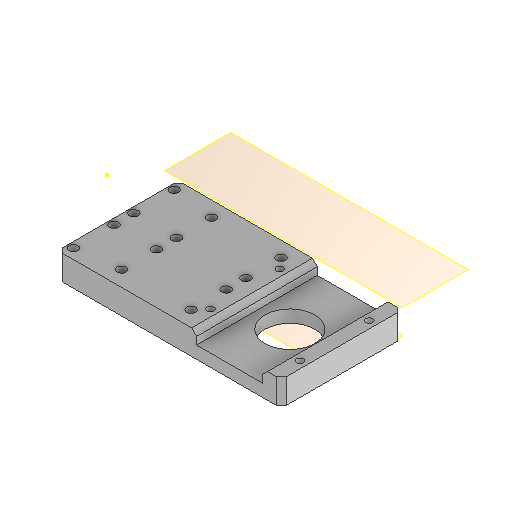
# Autodesk Inventor part: 60_Planktoscope_Sampleholder
Saved by Autodesk Inventor 2024.1 (Build 281209000, 209)
## iProperties
Created: 2024-03-06
Part Number: 60_Planktoscope_Sampleholder
Material: Generisch
Document SubType Name: Modeling
Designer: diederichbenedict
Density: 1 g/cm^3
Appearance: Vorgabe
Vendor: openUC2
Mass: 33.9876 g
Surface Area: 126.576 cm^2
Volume: 33.9876 cm^3
Author: diederichbenedict
Autodesk Inventor part; units mm, degrees
ref_plane "YZ Plane" through (0, 0, 0) normal (1, 0, 0) x (0, 1, 0)
ref_plane "XZ Plane" through (0, 0, 0) normal (0, 1, 0) x (-1, 0, 0)
ref_plane "XY Plane" through (0, 0, 0) normal (0, 0, 1) x (1, 0, 0)
ref_plane "Arbeitsebene1" through (0.2798, 48.6, 0) normal (0, 0, 1) x (1, 0, 0)
ref_plane "Arbeitsebene2" through (106.3244, 12.4, 0) normal (0, 0, 1) x (-1, 0, 0)
sketch "Skizze8" plane through (106.3244, 12.4, 0) normal (0, 0, 1) x (-1, 0, 0)
  circle A0 centre (8.6702, 4) radius 1.4 projected
  circle A1 centre (70.5201, 20.3) radius 1.4 projected
  circle A2 centre (8.6702, 20.3) radius 1.4 projected
  circle A3 centre (42.5201, 20.3) radius 1.4 projected
  circle A4 centre (42.5201, 6.2) radius 1.4 projected
  circle A5 centre (70.5201, 6.2) radius 1.4 projected
  circle A6 centre (87.6702, 20.3) radius 1.4 projected
  circle A7 centre (87.6702, 4) radius 1.4 projected
  line L0 (5, 0) -> (5, 24.3) projected
  line L1 (5, 0) -> (90, 0) projected
  line L2 (90, 24.3) -> (90, 0) projected
  line L3 (26.35, 24.3) -> (90, 24.3) projected
  arc A8 (15.35, 24.3) -> (26.35, 24.3) centre (20.85, 24.3) ccw projected
  line L4 (5, 24.3) -> (15.35, 24.3) projected
  circle A9 centre (8.6702, 44.6) radius 1.4 projected
  circle A10 centre (70.5201, 28.3) radius 1.4 projected
  circle A11 centre (8.6702, 28.3) radius 1.4 projected
  circle A12 centre (42.5201, 28.3) radius 1.4 projected
  circle A13 centre (42.5201, 42.4) radius 1.4 projected
  circle A14 centre (70.5201, 42.4) radius 1.4 projected
  circle A15 centre (87.6702, 28.3) radius 1.4 projected
  circle A16 centre (87.6702, 44.6) radius 1.4 projected
  line L5 (5, 48.6) -> (5, 24.3) projected
  line L6 (5, 24.3) -> (15.35, 24.3) projected
  arc A17 (26.35, 24.3) -> (15.35, 24.3) centre (20.85, 24.3) ccw projected
  line L7 (26.35, 24.3) -> (90, 24.3) projected
  line L8 (90, 24.3) -> (90, 48.6) projected
  line L9 (5, 48.6) -> (90, 48.6) projected
  line L10 (8.1, 62.05) -> (8.1, -13.45) projected
  circle A18 centre (20.85, 24.3) radius 10
  line L11 (5, 0) -> (0, 0)
  line L12 (0, 0) -> (0, 48.6)
  line L13 (0, 48.6) -> (5, 48.6)
  line L14 (5, 48.6) -> (5, 0)
  point P0 (106.3244, 12.4)
  point P1 (8.1, 48.6)
  point P2 (8.1, 45.8786)
  point P3 (8.1, 43.3214)
  point P4 (8.1, 29.5786)
  point P5 (8.1, 27.0214)
  point P6 (8.1, 21.5786)
  point P7 (8.1, 19.0214)
  point P8 (8.1, 5.2786)
  point P9 (8.1, 2.7214)
  point P10 (8.1, 0)
  dimension "d36" = 20
  dimension "d38" = 5
  constraints: 8 end point, 2 parallel, 1 centre point, 1 coincident, 1 horizontal, 1 perpendicular
  measures "d36" diameter of A18
  measures "d38" distance of L12.end L13.end
extrude "Extrusion6" add sketch "Skizze8" along normal blind 10 contours A0 L10 | A0 L10 A2 L4 A18 L3 L2 L1 | L10 A0 | A0 L10 L1 L0 L4 A2 | L10 A2 | A2 L10 | L11 L12 L13 L5 L0 | L10 A11 A9 L9 L8 L3 A18 L4 | L4 L5 L9 L10 A9 A11 | L10 A11 | A11 L10 | L10 A9 | A9 L10
sketch "Skizze9" plane through (106.3244, 12.4, 10) normal (0, 0, 1) x (1, 0, 0)
  arc A0 (-23.35, -48.1544) -> (-18.35, -48.1544) centre (-20.85, -49.3) ccw projected
  line L0 (-23.35, -48.1544) -> (-23.35, -0.4456) projected
  arc A1 (-18.35, -0.4456) -> (-23.35, -0.4456) centre (-20.85, 0.7) ccw projected
  line L1 (-18.35, -0.4456) -> (-18.35, -48.1544) projected
  line L2 (-33.6, 13.45) -> (-33.6, -62.05) projected
  line L3 (-33.6, -62.05) -> (-8.1, -62.05) projected
  line L4 (-8.1, -62.05) -> (-8.1, 13.45) projected
  line L5 (-8.1, 13.45) -> (-33.6, 13.45) projected
  line L6 (-34.1, -62.55) -> (-34.1, 13.95)
  line L7 (-34.1, 13.95) -> (-7.6, 13.95)
  line L8 (-7.6, 13.95) -> (-7.6, -62.55)
  line L9 (-7.6, -62.55) -> (-34.1, -62.55)
  point P0 (-106.3244, -12.4)
  dimension "d37" = 0.5
  constraints: 8 end point, 3 other
  measures "d37" distance between parallel lines of L2 L6
extrude "Extrusion7" cut sketch "Skizze9" against normal blind 5 contours L0 A1 L1 A0 | L5 L4 L3 L2 | L6 L7 L8 L9
chamfer "Fasen2" distance 2 angle 45 6 edges at (72.2244, -11.9, 10) (98.7244, -11.9, 10) (16.3244, -36.2, 5) (16.3244, 12.4, 5) (106.3244, 12.4, 5) (106.3244, -36.2, 5)
sketch "Skizze10" plane through (106.3244, 12.4, 10) normal (0, 0, 1) x (1, 0, 0)
  circle A0 centre (-87.6702, -44.6) radius 1.4 projected
  circle A1 centre (-70.5201, -42.4) radius 1.4 projected
  circle A2 centre (-42.5201, -28.3) radius 1.4 projected
  circle A3 centre (-70.5201, -28.3) radius 1.4 projected
  circle A4 centre (-42.5201, -42.4) radius 1.4 projected
  circle A5 centre (-87.6702, -28.3) radius 1.4 projected
  circle A6 centre (-70.5201, -20.3) radius 1.4 projected
  circle A7 centre (-42.5201, -20.3) radius 1.4 projected
  circle A8 centre (-42.5201, -6.2) radius 1.4 projected
  circle A9 centre (-70.5201, -6.2) radius 1.4 projected
  circle A10 centre (-87.6702, -20.3) radius 1.4 projected
  circle A11 centre (-87.6702, -4) radius 1.4 projected
  line L0 (-36.1, 0) -> (-36.1, -48.6) projected
  line L1 (-36.1, 0) -> (-88, 0) projected
  line L2 (-90, -2) -> (-90, -46.6) projected
  line L3 (-88, -48.6) -> (-36.1, -48.6) projected
  line L4 (-90, -2) -> (-88, 0) projected
  line L5 (-88, -48.6) -> (-90, -46.6) projected
  line L6 (0, -46.6) -> (-2, -48.6) projected
  line L7 (0, -46.6) -> (0, -2) projected
  line L8 (-2, 0) -> (0, -2) projected
  line L9 (-2, 0) -> (-5.6, 0) projected
  line L10 (-5.6, -48.6) -> (-5.6, 0) projected
  line L11 (-5.6, -48.6) -> (-2, -48.6) projected
  point P0 (-106.3244, -12.4)
  constraints: 11 coincident
hole "Bohrung3" at (18.6542, 8.4, 10) at (18.6542, -7.9, 10) at (18.6542, -32.2, 10) at (18.6542, -15.9, 10) at (35.8043, -15.9, 10) at (35.8043, -7.9, 10) at (35.8043, -30, 10) at (63.8043, -30, 10) at (63.8043, -15.9, 10) at (63.8043, -7.9, 10) at (63.8043, 6.2, 10) at (35.8043, 6.2, 10) direction (0, 0, -1) diameter 3.6 depth 15 tip angle 118
sketch "Skizze11" plane through (106.3244, 12.4, 10) normal (0, 0, 1) x (1, 0, 0)
  point P0 (-106.3244, -12.4)
sketch "Skizze12" plane through (106.3244, 12.4, 10) normal (0, 0, 1) x (1, 0, 0)
  circle A0 centre (-70.5201, -6.2) radius 1.8 projected
  circle A1 centre (-42.5201, -6.2) radius 1.8 projected
  circle A2 centre (-42.5201, -20.3) radius 1.8 projected
  circle A3 centre (-42.5201, -28.3) radius 1.8 projected
  circle A4 centre (-42.5201, -42.4) radius 1.8 projected
  circle A5 centre (-70.5201, -42.4) radius 1.8 projected
  circle A6 centre (-70.5201, -20.3) radius 1.8 projected
  circle A7 centre (-70.5201, -28.3) radius 1.8 projected
  circle A8 centre (-87.6702, -28.3) radius 1.8 projected
  circle A9 centre (-87.6702, -44.6) radius 1.8 projected
  circle A10 centre (-87.6702, -20.3) radius 1.8 projected
  circle A11 centre (-87.6702, -4) radius 1.8 projected
  line L0 (-36.1, 0) -> (-36.1, -48.6) projected
  line L1 (-36.1, 0) -> (-88, 0) projected
  line L2 (-90, -2) -> (-90, -46.6) projected
  line L3 (-88, -48.6) -> (-36.1, -48.6) projected
  circle A12 centre (-20.85, -24.3) radius 10 projected
  line L4 (-38.85, -38.3) -> (-2.85, -38.3)
  line L5 (-2.85, -38.3) -> (-2.85, -10.3)
  line L6 (-2.85, -10.3) -> (-38.85, -10.3)
  line L7 (-38.85, -10.3) -> (-38.85, -38.3)
  line L8 (-38.85, -38.3) -> (-2.85, -10.3) construction
  line L9 (-2.85, -38.3) -> (-38.85, -10.3) construction
  line L10 (-90, -2) -> (-88, 0) projected
  line L11 (-88, -48.6) -> (-90, -46.6) projected
  line L12 (0, -46.6) -> (-2, -48.6) projected
  line L13 (0, -46.6) -> (0, -2) projected
  line L14 (-2, 0) -> (0, -2) projected
  line L15 (-2, 0) -> (-5.6, 0) projected
  line L16 (-5.6, -48.6) -> (-5.6, 0) projected
  line L17 (-5.6, -48.6) -> (-2, -48.6) projected
  point P0 (-106.3244, -12.4)
  dimension "d51" = 36
  dimension "d52" = 28
  constraints: 12 end point, 2 midpoint, 2 parallel, 1 horizontal, 1 perpendicular
  measures "d51" distance of L6.end L5.end
  measures "d52" distance of L5.end L4.end
hole "Bohrung4" at (67.4744, 2.1, 10) at (67.4744, -25.9, 10) at (103.4744, 2.1, 10) at (103.4744, -25.9, 10) direction (0, 0, -1) diameter 2.8 depth 15 tip angle 118
